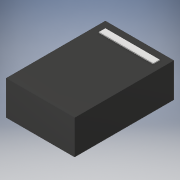
# Autodesk Inventor part: Semiconductor_UDFN-6
Saved by Autodesk Inventor 2018 (Build 220112000, 112)
## iProperties
Created: 2016-07-11
Part Number: Semiconductor_UDFN-6
Material: ABS Plastic
Document SubType Name: Modeling
Designer: Bradley
Density: 1.06 g/cm^3
Appearance: Smooth - Black
Author: Bradley
Autodesk Inventor part; units mm, degrees
ref_plane "YZ Plane" through (0, 0, 0) normal (1, 0, 0) x (0, 1, 0)
ref_plane "XZ Plane" through (0, 0, 0) normal (0, 1, 0) x (-1, 0, 0)
ref_plane "XY Plane" through (0, 0, 0) normal (0, 0, 1) x (1, 0, 0)
sketch "Sketch1" plane through (0, 0, 0) normal (0, 1, 0) x (-1, 0, 0)
  line L0 (-0.5, 0.725) -> (0.5, 0.725)
  line L1 (0.5, 0.725) -> (0.5, -0.725)
  line L2 (0.5, -0.725) -> (-0.5, -0.725)
  line L3 (-0.5, -0.725) -> (-0.5, 0.725)
  line L4 (-0.5, 0.725) -> (0.5, -0.725) construction
  line L5 (0.5, 0.725) -> (-0.5, -0.725) construction
  point P0 (0, 0)
  dimension "d0" = 1
  dimension "d1" = 1.45
  constraints: 12 end point, 2 midpoint, 2 parallel, 1 horizontal, 1 perpendicular
  measures "d0" distance of L1.end L2.end
  measures "d1" distance of L0.end L1.end
extrude "Extrusion1" add sketch "Sketch1" along normal mid plane 0.5
sketch "Sketch2" plane through (0, -0.25, 0) normal (0, -1, 0) x (1, 0, 0)
  line L0 (0.5, 0.725) -> (-0.5, 0.725) projected
  line L1 (-0.5, 0.725) -> (-0.5, -0.725) projected
  line L2 (-0.5, -0.725) -> (0.5, -0.725) projected
  line L3 (0.5, -0.725) -> (0.5, 0.725) projected
  line L4 (0.5, -0.725) -> (-0.5, -0.725) projected
  line L5 (0.5, 0.725) -> (0.5, -0.725) projected
  line L6 (0.45, -0.6) -> (0.15, -0.6)
  line L7 (0.15, -0.6) -> (0.15, -0.4)
  line L8 (0.15, -0.4) -> (0.45, -0.4)
  line L9 (0.45, -0.4) -> (0.45, -0.6)
  line L10 (-0.5, 0.725) -> (0.5, 0.725) projected
  line L11 (-0.5, -0.725) -> (-0.5, 0.725) projected
  line L12 (-0.45, -0.6) -> (-0.15, -0.6)
  line L13 (-0.15, -0.6) -> (-0.15, -0.4)
  line L14 (-0.15, -0.4) -> (-0.45, -0.4)
  line L15 (-0.45, -0.4) -> (-0.45, -0.6)
  line L16 (0.45, -0.1) -> (0.15, -0.1)
  line L17 (0.15, -0.1) -> (0.15, 0.1)
  line L18 (0.15, 0.1) -> (0.45, 0.1)
  line L19 (0.45, 0.1) -> (0.45, -0.1)
  line L20 (-0.45, -0.1) -> (-0.15, -0.1)
  line L21 (-0.45, 0.1) -> (-0.45, -0.1)
  line L22 (-0.15, 0.1) -> (-0.45, 0.1)
  line L23 (-0.15, -0.1) -> (-0.15, 0.1)
  line L24 (0.45, 0.4) -> (0.15, 0.4)
  line L25 (0.15, 0.4) -> (0.15, 0.6)
  line L26 (0.15, 0.6) -> (0.45, 0.6)
  line L27 (0.45, 0.6) -> (0.45, 0.4)
  line L28 (-0.45, 0.4) -> (-0.15, 0.4)
  line L29 (-0.45, 0.6) -> (-0.45, 0.4)
  line L30 (-0.15, 0.6) -> (-0.45, 0.6)
  line L31 (-0.15, 0.4) -> (-0.15, 0.6)
  point P0 (0, 0)
  point P1 (0.5, 0)
  dimension "d8" = 0.3
  dimension "d9" = 0.2
  dimension "d20" = 0.5
  dimension "d71" = 0.35
  dimension "d72" = 0.35
  constraints: 48 end point, 4 parallel, 2 equal length, 2 horizontal, 2 perpendicular, 1 collinear, 1 midpoint, 1 vertical, 32 other
  measures "d8" distance of L6.start L6.end
  measures "d9" distance of L6.end L7.end
  measures "d20" distance of L6.start L16.start
  measures "d71" distance between parallel lines of L7 L3
  measures "d72" distance between parallel lines of L13 L1
extrude "Extrusion2" add sketch "Sketch2" along normal blind 0.035 contours L6 L7 L8 L9 | L15 L14 L13 L12 | L16 L17 L18 L19 | L21 L22 L23 L20 | L24 L25 L26 L27 | L29 L30 L31 L28
sketch "Sketch5" plane through (0, 0.25, 0) normal (0, 1, 0) x (1, 0, 0)
  line L0 (-0.5, -0.725) -> (0.5, -0.725) projected
  line L1 (0.5, -0.725) -> (0.5, 0.725) projected
  line L2 (0.5, 0.725) -> (-0.5, 0.725) projected
  line L3 (-0.5, 0.725) -> (-0.5, -0.725) projected
  line L4 (-0.5, 0.725) -> (-0.5, -0.725) construction
  line L5 (0.4, 0.625) -> (-0.4, 0.625)
  line L6 (-0.4, 0.625) -> (-0.4, 0.525)
  line L7 (-0.4, 0.525) -> (0.4, 0.525)
  line L8 (0.4, 0.525) -> (0.4, 0.625)
  circle A0 centre (-0.4, 0.625) radius 0.1 construction
  point P0 (0, 0.525)
  point P1 (0, 0.725)
  dimension "d73" = 0.8
  dimension "d74" = 0.1
  constraints: 8 end point, 2 midpoint, 2 parallel, 2 tangent, 1 centre point, 1 coincident, 1 horizontal, 1 perpendicular, 1 vertical alignment
  measures "d73" distance of L7.end L6.end
  measures "d74" distance of L7.end L5.start
extrude "Extrusion5" add sketch "Sketch5" along normal blind 0.01 contours L8 L7 L6 L5
equation "\"d72\" = d71"
body "Solid1"
